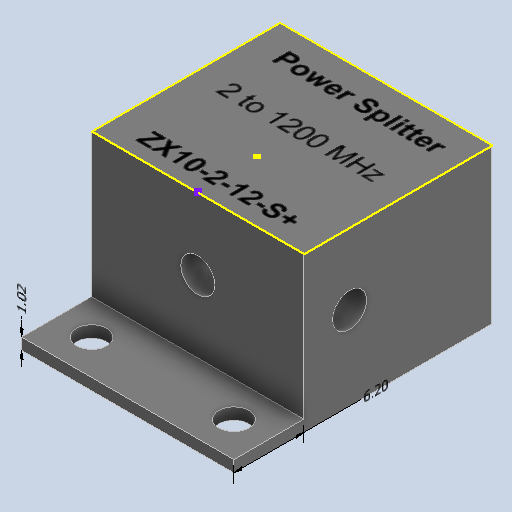
# Autodesk Inventor part: ZX10-2-12-S+
Saved by Autodesk Inventor 2024 (Build 280153000, 153)
## iProperties
Created: 2023-10-01
Part Number: ZX10-2-12-S+
Material: Generic
Document SubType Name: Modeling
Designer: Alexander Pollak
Density: 1 g/cm^3
Appearance: Gray
Author: Alexander Pollak
Autodesk Inventor part; units mm, degrees
ref_plane "YZ Plane" through (0, 0, 0) normal (1, 0, 0) x (0, 1, 0)
ref_plane "XZ Plane" through (0, 0, 0) normal (0, 1, 0) x (-1, 0, 0)
ref_plane "XY Plane" through (0, 0, 0) normal (0, 0, 1) x (1, 0, 0)
sketch "mounting sheet" plane through (0, 0, 0) normal (0, 1, 0) x (-1, 0, 0)
  line L0 (9.4, -11.43) -> (-9.4, -11.43)
  line L1 (-9.4, -11.43) -> (-9.4, 11.43)
  line L2 (-9.4, 11.43) -> (9.4, 11.43)
  line L3 (9.4, 11.43) -> (9.4, -11.43)
  line L4 (9.4, -11.43) -> (-9.4, 11.43) construction
  line L5 (-9.4, -11.43) -> (9.4, 11.43) construction
  point P0 (0, 0)
  dimension "d0" = 18.8
  dimension "d1" = 22.86
  constraints: 12 end point, 2 midpoint, 2 parallel, 1 horizontal, 1 perpendicular
  measures "d0" distance of L1.end L2.end
  measures "d1" distance of L0.end L1.end
extrude "mounting" add sketch "mounting sheet" along normal blind 1.02
sketch "Sketch2" plane through (0, 1.02, 0) normal (0, 1, 0) x (1, 0, 0)
  line L0 (-9.4, 11.43) -> (-9.4, -11.43) construction
  line L1 (-9.4, -8.33) -> (9.4, -8.33) construction
  line L2 (9.4, -11.43) -> (9.4, 11.43) construction
  line L3 (-9.4, -11.43) -> (9.4, -11.43) construction
  point P0 (0, 0)
  point P1 (-6.3, -8.33)
  point P2 (6.3, -8.33)
  dimension "d10" = 3.1
  dimension "d11" = 3.1
  dimension "d12" = 12.6
  constraints: 4 point on line, 2 end point, 1 horizontal
  measures "d10" distance between parallel lines of L3 L1
  measures "d11" distance from line of point (-6.3, -8.33) L0
  measures "d12" distance of point (6.3, -8.33) point (-6.3, -8.33)
hole "Hole1" at (-6.3, 1.02, 8.33) at (6.3, 1.02, 8.33) direction (0, -1, 0) diameter 2.69 end through all
sketch "Sketch4" plane through (0, 1.02, 0) normal (0, 1, 0) x (1, 0, 0)
  line L0 (9.4, 11.43) -> (-9.4, 11.43) projected
  line L1 (9.4, -11.43) -> (9.4, 11.43) projected
  line L2 (-9.4, 11.43) -> (9.4, 11.43)
  line L3 (9.4, 11.43) -> (9.4, -5.23)
  line L4 (9.4, -5.23) -> (-9.4, -5.23)
  line L5 (-9.4, -5.23) -> (-9.4, 11.43)
  line L6 (-9.4, -11.43) -> (9.4, -11.43) projected
  point P0 (0, 0)
  dimension "d21" = 6.2
  constraints: 8 end point, 2 parallel, 1 horizontal, 1 perpendicular, 1 point on line
  measures "d21" distance between parallel lines of L4 L6
extrude "Extrusion2" add sketch "Sketch4" along normal blind 12.7
sketch "Sketch5" plane through (-9.4, 1.02, 5.23) normal (0, 0, 1) x (1, 0, 0)
  line L0 (18.8, 12.7) -> (0, 12.7) construction
  line L1 (9.4, 12.7) -> (9.4, 0) construction
  line L2 (0, 0) -> (18.8, 0) construction
  line L3 (18.8, -1.02) -> (18.8, 12.7) construction
  line L4 (0, -1.02) -> (0, 12.7) construction
  line L5 (18.8, 6.35) -> (0, 6.35) construction
  point P0 (9.4, -1.02)
  point P1 (9.4, 6.35)
  dimension "d25" = 7.37
  constraints: 4 end point, 3 midpoint, 2 point on line, 1 perpendicular
  measures "d25" distance from line of L3.start L5
hole "Hole2" at (0, 7.37, 5.23) direction (0, 0, -1) diameter 3 depth 5 tip angle 118
sketch "Sketch6" plane through (9.4, 0, 11.43) normal (1, 0, 0) x (0, 0, -1)
  line L0 (6.2, 1.02) -> (6.2, 13.72) construction
  line L1 (6.2, 7.37) -> (22.8459, 7.37) construction
  line L2 (6.2, 13.72) -> (22.86, 13.72) construction
  line L3 (0, 0) -> (22.86, 0) construction
  line L4 (10.26, 13.72) -> (10.26, 0) construction
  point P0 (11.43, 0)
  point P1 (10.26, 7.37)
  dimension "d33" = 4.06
  dimension "d34" = 7.37
  constraints: 4 end point, 4 point on line, 1 horizontal, 1 midpoint, 1 perpendicular
  measures "d33" distance between parallel lines of L0 L4
  measures "d34" distance between parallel lines of L3 L1
hole "Hole3" at (9.4, 7.37, 1.17) direction (-1, 0, 0) diameter 3 end through all
sketch "Sketch7" plane through (0, 13.72, 0) normal (0, 1, 0) x (1, 0, 0)
  line L0 (-9.4, 11.43) -> (9.4, 11.43) construction
  line L1 (9.4, 11.43) -> (9.4, -5.23) construction
  line L2 (9.4, -5.23) -> (-9.4, -5.23) construction
  line L3 (-9.4, -5.23) -> (-9.4, 11.43) construction
  line L4 (-9.4, 11.43) -> (-9.4, -5.23) projected
  line L5 (9.4, -5.23) -> (9.4, 11.43) projected
  line L6 (9.4, 11.43) -> (-9.4, 11.43) projected
  line L7 (-9.4, -5.23) -> (9.4, -5.23) projected
  point P0 (0, 0)
  point P1 (0, -5.23)
  constraints: 1 midpoint, 2 other
